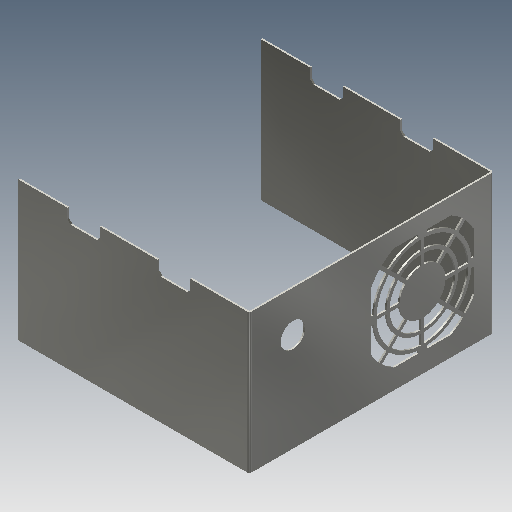
# Autodesk Inventor part: config - power supply - back casing
Saved by Autodesk Inventor 2020 (Build 240152000, 152)
## iProperties
Created: 2005-12-21
Part Number: config - power supply - back casing
Material: Generic
Document SubType Name: Sheet Metal
Designer: Simon.Ng@autodesk.com
Stock Number: config - power supply - back casing
Density: 1 g/cm^3
Sheet Metal Rule: 1.0 mm
Mass: 33.4585 g
Surface Area: 691.144 cm^2
Volume: 33.4585 cm^3
Appearance: Silicon Nitride - Polished
Company: Autodesk Asia Pte. Ltd.
Title: PC Demo
Author: Simon.Ng@autodesk.com
Autodesk Inventor part; units mm, degrees
ref_plane "YZ Plane" through (0, 0, 0) normal (1, 0, 0) x (0, 1, 0)
ref_plane "XZ Plane" through (0, 0, 0) normal (0, 1, 0) x (-1, 0, 0)
ref_plane "XY Plane" through (0, 0, 0) normal (0, 0, 1) x (1, 0, 0)
sketch "Sketch3" plane through (0, 0, 0) normal (1, 0, 0) x (0, 1, 0)
  line L0 (85, 150) -> (0, 150)
  line L1 (0, 150) -> (0, 0)
  line L2 (85, 0) -> (85, 150)
  line L3 (0, 149) -> (85, 149)
  line L4 (0, 149) -> (85, 149)
  line L5 (85, 149) -> (85, 0)
  line L6 (85, 0) -> (0, 0)
  line L7 (0, 0) -> (0, 149)
  dimension "d52" = 1
  measures "d52" distance between parallel lines of L0 L3
extrude "Plate1" add sketch "Sketch3" against normal blind 1 contours L2 L6 L1 L3
sketch "Sketch4" plane through (0, 0, 149) normal (0, 0, -1) x (0, 1, 0)
  line L0 (0, 0) -> (85, 0)
  line L1 (85, 0) -> (85, -141)
  line L2 (85, -141) -> (0, -141)
  line L3 (0, -141) -> (0, 0)
  constraints: 4 end point, 4 other
sheet face with bend "Flange1" sketch "Sketch4" thickness 1 toward (0, 0, -1) bend radius 0.5 relief round relief width 1 relief depth 0.5
bend "Bend1"
sketch "Sketch5" plane through (0, 85, 0) normal (0, 0, 1) x (0, -1, 0)
  line L0 (0, 0) -> (85, 0)
  line L1 (85, 0) -> (85, -141)
  line L2 (85, -141) -> (0, -141)
  line L3 (0, -141) -> (0, 0)
  constraints: 4 end point, 4 other
sheet face with bend "Flange2" sketch "Sketch5" thickness 1 toward (0, 0, 1) bend radius 0.5 relief round relief width 1 relief depth 0.5
bend "Bend2"
sketch "Sketch6" plane through (-141, 0, 0) normal (0, 0, -1) x (-1, 0, 0)
  line L0 (0, 0) -> (0, 85) projected
  line L1 (0, 85) -> (-139.5, 85) projected
  line L2 (-105, 85) -> (-85, 85)
  line L3 (-85, 85) -> (-85, 77)
  line L4 (-85, 77) -> (-105, 77)
  line L5 (-105, 77) -> (-105, 85)
  line L6 (-50, 85) -> (-30, 85)
  line L7 (-30, 85) -> (-30, 77)
  line L8 (-30, 77) -> (-50, 77)
  line L9 (-50, 77) -> (-50, 85)
  dimension "d17" = 30
  dimension "d18" = 35
  dimension "d19" = 8
  dimension "d20" = 20
  constraints: 16 end point, 4 parallel, 2 collinear, 2 horizontal, 2 perpendicular, 2 point on line
  measures "d17" distance between parallel lines of L0 L7
  measures "d18" distance between parallel lines of L9 L3
  measures "d19" distance of L6.end L7.end
  measures "d20" distance of L7.end L8.end
extrude "Cut1" cut sketch "Sketch6" against normal blind 1
chamfer "Corner Chamfer1" distance 2 angle 45 4 edges at (-36, 77, 0.5) (-56, 77, 0.5) (-91, 77, 0.5) (-111, 77, 0.5)
ref_plane "Work Plane1" through (-141, 0, 74.5) normal (0, 0, -1) x (-1, 0, 0)
mirror "Mirror2" about plane through (-141, 0, 74.5) normal (0, 0, -1) of "Cut1", "Corner Chamfer1"
sketch "Sketch8" plane through (0, 0, 147.5) normal (1, 0, 0) x (0, 1, 0)
  circle A0 centre (60, -25) radius 7.5
  line L0 (85, -146) -> (85, 0) projected
  line L1 (85, 0) -> (0, 0) projected
  dimension "d74" = 15
  dimension "d75" = 25
  dimension "d76" = 25
  constraints: 1 centre point
  measures "d74" diameter of A0
  measures "d75" distance from line of L0 A0.centre
  measures "d76" distance from line of L1 A0.centre
extrude "Cut3" cut sketch "Sketch8" against normal blind 1
sketch "Sketch9" plane through (0, 0, 147.5) normal (1, 0, 0) x (0, 1, 0)
  line L0 (85, -146) -> (85, 0) projected
  line L1 (12, -72.5) -> (75, -72.5) construction
  line L2 (75, -72.5) -> (75, -135.5) construction
  line L3 (75, -135.5) -> (12, -135.5) construction
  line L4 (12, -135.5) -> (12, -72.5) construction
  line L5 (0, -147.5) -> (85, -147.5) projected
  line L6 (43.5, -72.5) -> (43.5, -135.5) construction
  line L7 (12, -104) -> (75, -104) construction
  line L8 (43.5, -104) -> (75, -72.5) construction
  line L9 (42.5, -104) -> (44.5, -104) construction
  line L10 (44.5, -104) -> (44.5, -72.5) construction
  line L11 (44.5, -72.5) -> (42.5, -72.5) construction
  line L12 (42.5, -72.5) -> (42.5, -104) construction
  line L13 (43.5, -103) -> (75, -103) construction
  line L14 (75, -103) -> (75, -105) construction
  line L15 (75, -105) -> (43.5, -105) construction
  line L16 (43.5, -105) -> (43.5, -103) construction
  line L17 (37.8783, -108.2075) -> (74.2929, -71.7929) construction
  line L18 (74.2929, -71.7929) -> (75.7071, -73.2071) construction
  line L19 (75.7071, -73.2071) -> (39.2925, -109.6217) construction
  line L20 (39.2925, -109.6217) -> (37.8783, -108.2075) construction
  circle A0 centre (43.5, -104) radius 14 construction
  circle A1 centre (43.5, -104) radius 20 construction
  circle A2 centre (43.5, -104) radius 22 construction
  circle A3 centre (43.5, -104) radius 28 construction
  circle A4 centre (43.5, -104) radius 30 construction
  line L21 (46, -74.1043) -> (46, -72.5)
  arc A5 (68.2389, -77.8469) -> (60.9284, -72.5) centre (43.5, -104) ccw
  line L22 (46, -72.5) -> (60.9284, -72.5)
  line L23 (68.2389, -77.8469) -> (63.9943, -82.0915)
  line L24 (62.5793, -83.5065) -> (58.3332, -87.7526)
  line L25 (56.9173, -89.1684) -> (52.6671, -93.4187)
  line L26 (44.5, -90.0358) -> (44.5, -84.025)
  line L27 (44.5, -82.0227) -> (44.5, -76.0179)
  arc A6 (52.6671, -93.4187) -> (44.5, -90.0358) centre (43.5, -104) ccw
  arc A7 (56.9173, -89.1684) -> (44.5, -84.025) centre (43.5, -104) ccw
  arc A8 (58.3332, -87.7526) -> (44.5, -82.0227) centre (43.5, -104) ccw
  arc A9 (62.5793, -83.5065) -> (44.5, -76.0179) centre (43.5, -104) ccw
  arc A10 (63.9943, -82.0915) -> (46, -74.1043) centre (43.5, -104) ccw
  line L28 (44.5, -84.025) -> (44.5, -90.0358)
  line L29 (56.9173, -89.1684) -> (52.6671, -93.4187)
  dimension "d54" = 63
  dimension "d55" = 10
  dimension "d56" = 12
  dimension "d57" = 2
  dimension "d58" = 2
  dimension "d59" = 28
  dimension "d60" = 2
  dimension "d61" = 40
  dimension "d62" = 2
  dimension "d63" = 56
  dimension "d64" = 2.5
  dimension "d65" = 36
  dimension "d66" = 6
  dimension "d67" = 6
  constraints: 56 end point, 22 point on circle, 16 point on line, 11 centre point, 11 coincident, 9 parallel, 7 perpendicular, 6 midpoint, 3 collinear, 3 horizontal, 2 other
  measures "d54" distance of L1.end L2.end
  measures "d55" distance between parallel lines of L0 L2
  measures "d56" distance between parallel lines of L5 L3
  measures "d57" distance between parallel lines of L12 L10
  measures "d58" distance of L19.end L17.start
  measures "d59" diameter of A0
  measures "d60" radial gap between concentric circles of A2 A1
  measures "d61" diameter of A1
  measures "d62" radial gap between concentric circles of A4 A3
  measures "d63" diameter of A3
  measures "d64" distance between parallel lines of L6 L21
  measures "d65" radius of A5
  measures "d66" radial gap between concentric circles of A2 A3
  measures "d67" radial gap between concentric circles of A0 A1
extrude "Cut4" cut sketch "Sketch9" against normal blind 1
ref_plane "Work Plane3" through (0, 43.5, 43.5) normal (0, 0.7071068, -0.7071068) x (0, 0.7071068, 0.7071068)
mirror "Mirror4" about plane through (0, 43.5, 43.5) normal (0, 0.7071068, -0.7071068) of "Cut4"
pattern_circular "Circular Pattern2" count 4 over 360 about axis through (0, 43.5, 43.5) along (1, 0, 0) of "Cut4", "Mirror4"
equation "\"d21\" = Thickness"
equation "\"d49\" = Thickness"
equation "\"d60\" = d57"
equation "\"d62\" = d60"
equation "\"d68\" = Thickness"
equation "\"d77\" = Thickness"
equation "\"d4\" = MinimumRemnant"
equation "\"d8\" = BendRadius"
equation "\"d2\" = BendReliefWidth"
equation "\"d3\" = BendReliefDepth"
equation "\"d5\" = BendRadius"
equation "\"d11\" = MinimumRemnant"
equation "\"d15\" = BendRadius"
equation "\"d9\" = BendReliefWidth"
equation "\"d10\" = BendReliefDepth"
equation "\"d12\" = BendRadius"
equation "\"BendReliefWidth\" = Thickness"
equation "\"BendReliefDepth\" = 0.5 * Thickness"
equation "\"CornerReliefSize\" = 4 * Thickness"
equation "\"MinimumRemnant\" = 2 * Thickness"
equation "\"TransitionRadius\" = BendRadius"
equation "\"d16\" = 142"
equation "\"d1\" = BendRadius"
equation "\"JacobiRadiusSize\" = Thickness"
equation "\"GapSize\" = Thickness"
equation "\"Thickness\" = 1"
equation "\"BendRadius\" = 0.5"
body "Solid1"
